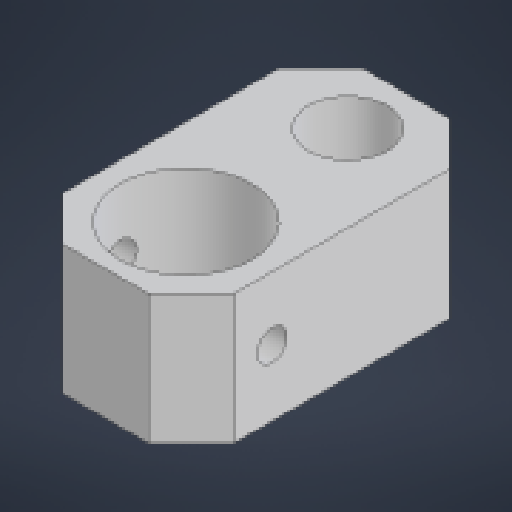
# Autodesk Inventor part: Z axis collar
Saved by Autodesk Inventor 2026 (Build 300175050, 175E)
## iProperties
Created: 2025-07-01
Part Number: Z axis collar
Material: Generic
Document SubType Name: Modeling
Designer: Tobymegacat
Density: 1 g/cm^3
Appearance: Default
Author: Tobymegacat
Autodesk Inventor part; units mm, degrees
ref_plane "YZ Plane" through (0, 0, 0) normal (1, 0, 0) x (0, 1, 0)
ref_plane "XZ Plane" through (0, 0, 0) normal (0, 1, 0) x (-1, 0, 0)
ref_plane "XY Plane" through (0, 0, 0) normal (0, 0, 1) x (1, 0, 0)
sketch "Sketch1" plane through (0, 0, 0) normal (0, 1, 0) x (-1, 0, 0)
  circle A0 centre (0, 0) radius 6.1
  circle A1 centre (0, -15) radius 3.65
  line L0 (8, 7.5) -> (-8, 7.5)
  line L1 (-8, 7.5) -> (-8, -20.5)
  line L2 (-8, -20.5) -> (8, -20.5)
  line L3 (8, -20.5) -> (8, 7.5)
  dimension "d0" = 12.2
  dimension "d1" = 7.3
  dimension "d2" = 15
  dimension "d3" = 16
  dimension "d4" = 8
  dimension "d5" = 28
  dimension "d6" = 5.5
  constraints: 8 end point, 2 centre point, 2 parallel, 1 coincident, 1 horizontal, 1 perpendicular
  measures "d0" diameter of A0
  measures "d1" diameter of A1
  measures "d2" distance of point (0, 0) A1.centre
  measures "d3" distance of L1.end L2.end
  measures "d4" distance from line of L3 point (0, 0)
  measures "d5" distance of L0.end L1.end
  measures "d6" distance from line of L2 A1.centre
extrude "Extrusion1" add sketch "Sketch1" along normal blind 12
chamfer "Chamfer1" distance 4 angle 45 4 edges at (8, 6, -20.5) (-8, 6, -20.5) (8, 6, 7.5) (-8, 6, 7.5)
sketch "Sketch3" plane through (8, 0, 3.5) normal (1, 0, 0) x (0, 0, -1)
  line L0 (-4, 12) -> (-4, 0) projected
  point P0 (3.5, 0)
  point P1 (3.5, 6.0888)
  dimension "d12" = 7.5
  measures "d12" distance from line of L0 point (3.5, 6.089)
hole "Hole1" at (8, 6.0888, 0) direction (-1, 0, 0) diameter 2.8 depth 17.75
sketch "Sketch4" plane through (4, 0, -20.5) normal (0, 0, -1) x (-1, 0, 0)
  line L0 (8, 12) -> (8, 0) projected
  line L1 (0, 0) -> (8, 0) projected
  point P0 (4, 0)
  point P1 (4, 6.1062)
  dimension "d20" = 4
  dimension "d21" = 6.1062
  measures "d20" distance from line of L0 point (4, 6.106)
  measures "d21" distance from line of L1 point (4, 6.106)
hole "Hole2" at (0, 6.1062, -20.5) direction (0, 0, 1) diameter 2.8 depth 5
body "Solid1"
